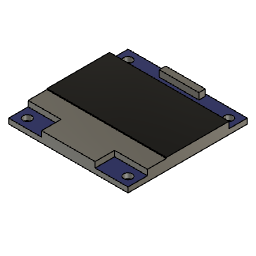
Enclosure_2_v72 (Autodesk Fusion 360 archive; units mm, degrees)
design "OLED"
Autodesk Fusion 360 part; units mm, degrees
sketch "Sketch1" plane through (0, 0, 0) normal (0, 0, 1) x (1, 0, 0)
  line L0 (0, 0) -> (27.85, 0)
  line L1 (27.85, 0) -> (27.85, 27.85)
  line L2 (27.85, 27.85) -> (0, 27.85)
  line L3 (0, 27.85) -> (0, 0)
  dimension "d1" = 27.85
  dimension "d2" = 27.85
  constraint horizontal L0
  constraint vertical L1
  constraint horizontal L2
  constraint vertical L3
  constraint coincident L0.start L3.end
  measures "d1" distance of L0.start L0.end
  measures "d2" distance of L0.start L2.end
extrude "Extrude1" add sketch "Sketch1" along normal blind 1.2
sketch "Sketch2" plane through (0, 0, 1.2) normal (0, 0, 1) x (-1, 0, 0)
  line L0 (0, -27.85) -> (0, 0)
  line L1 (0, 0) -> (-27.85, 0)
  line L2 (-27.85, 0) -> (-27.85, -27.85)
  line L3 (-27.85, -27.85) -> (0, -27.85)
  circle A0 centre (-2.175, -25.675) radius 1
  circle A1 centre (-2.175, -2.175) radius 1
  circle A2 centre (-25.675, -25.675) radius 1
  circle A3 centre (-25.675, -2.175) radius 1
  line L4 (0, -24.675) -> (-27.85, -24.675) construction
  line L5 (0, -3.175) -> (-27.85, -3.175) construction
  line L6 (-24.675, 0) -> (-24.675, -27.85) construction
  line L7 (-3.175, 0) -> (-3.175, -27.85) construction
  line L8 (-24.675, -13.925) -> (-27.85, -13.925) construction
  line L9 (-3.175, -13.925) -> (0, -13.925) construction
  line L10 (-13.925, -24.675) -> (-13.925, -27.85) construction
  line L11 (-13.925, -3.175) -> (-13.925, 0) construction
  dimension "d5" = 2
  dimension "d6" = 21.5
  dimension "d7" = 21.5
  constraint coincident L0 L4.start
  constraint coincident L2 L4.end
  constraint perpendicular L2 L4
  constraint coincident L0 L5.start
  constraint coincident L2 L5.end
  constraint perpendicular L2 L5
  constraint coincident L1 L6.start
  constraint coincident L3 L6.end
  constraint perpendicular L3 L6
  constraint coincident L1 L7.start
  constraint coincident L3 L7.end
  constraint perpendicular L3 L7
  constraint equal A0 A2
  constraint equal A0 A1
  constraint equal A0 A3
  constraint tangent A0 L4
  constraint tangent A0 L7
  constraint tangent A1 L7
  constraint tangent A1 L5
  constraint tangent A3 L5
  constraint tangent A3 L6
  constraint tangent A2 L4
  constraint tangent A2 L6
  constraint midpoint L6 L8.start
  constraint midpoint L2 L8.end
  constraint midpoint L7 L9.start
  constraint midpoint L0 L9.end
  constraint midpoint L4 L10.start
  constraint midpoint L3 L10.end
  constraint midpoint L5 L11.start
  constraint midpoint L1 L11.end
  constraint equal L8 L9
  constraint equal L10 L11
  measures "d5" diameter of A0
  measures "d6" distance of L4 L5
  measures "d7" distance of L6 L7
extrude "Extrude2" cut sketch "Sketch2" against normal through all contours A0 | A1 | A2 | A3
sketch "Sketch3" plane through (0, 0, 1.2) normal (0, 0, 1) x (-1, 0, 0)
  circle A0 centre (-25.675, -2.175) radius 1
  circle A1 centre (-25.675, -25.675) radius 1
  circle A2 centre (-2.175, -2.175) radius 1
  circle A3 centre (-2.175, -25.675) radius 1
  line L0 (0, -27.85) -> (0, 0)
  line L1 (0, 0) -> (-27.85, 0)
  line L2 (-27.85, 0) -> (-27.85, -27.85)
  line L3 (-27.85, -27.85) -> (0, -27.85)
  line L4 (0, -23.55) -> (-27.85, -23.55)
  line L5 (-27.85, -23.55) -> (-27.85, -4.55)
  line L6 (-27.85, -4.55) -> (0, -4.55)
  line L7 (0, -4.55) -> (0, -23.55)
  line L8 (-7.675, -4.55) -> (-20.175, -4.55)
  line L9 (-20.175, -4.55) -> (-20.175, 0)
  line L10 (-20.175, 0) -> (-7.675, 0)
  line L11 (-7.675, 0) -> (-7.675, -4.55)
  line L12 (-13.925, 0) -> (-13.925, -4.55) construction
  dimension "d9" = 19
  dimension "d10" = 4.3
  dimension "d13" = 12.5
  constraint horizontal L4
  constraint vertical L5
  constraint horizontal L6
  constraint vertical L7
  constraint coincident L2 L5.end
  constraint coincident L0 L4.start
  constraint horizontal L8
  constraint vertical L9
  constraint horizontal L10
  constraint vertical L11
  constraint coincident L1 L9.end
  constraint coincident L6 L8.start
  constraint midpoint L10 L12.start
  constraint midpoint L6 L12.end
  constraint vertical L12
  measures "d9" distance of L4 L6
  measures "d10" distance of L3 L4
  measures "d13" distance of L9.end L10.end
extrude "Extrude3" add sketch "Sketch3" along normal blind 1.5 contours L0 L2 L4 L5 L6 L7 L8
extrude "Extrude4" add sketch "Sketch3" along normal blind 1.3 contours L1 L6 L8 L9 L10 L11
sketch "Sketch4" plane through (0, 0, 1.2) normal (0, 0, 1) x (-1, 0, 0)
  line L0 (0, -23.55) -> (-27.85, -23.55)
  line L1 (-27.85, -23.55) -> (-27.85, -27.85)
  line L2 (-27.85, -27.85) -> (0, -27.85)
  line L3 (0, -27.85) -> (0, -23.55)
  circle A0 centre (-25.675, -25.675) radius 1
  circle A1 centre (-2.175, -25.675) radius 1
  line L4 (-9.3, -27.35) -> (-18.55, -27.35)
  line L5 (-18.55, -27.35) -> (-18.55, -25.85)
  line L6 (-18.55, -25.85) -> (-9.3, -25.85)
  line L7 (-9.3, -25.85) -> (-9.3, -27.35)
  line L8 (-13.925, -27.85) -> (-13.925, -27.35) construction
  dimension "d16" = 2
  dimension "d17" = 1.5
  dimension "d18" = 9.25
  constraint horizontal L4
  constraint vertical L5
  constraint horizontal L6
  constraint vertical L7
  constraint midpoint L2 L8.start
  constraint midpoint L4 L8.end
  constraint vertical L8
  measures "d16" distance of L2 L6
  measures "d17" distance of L4.start L6.end
  measures "d18" distance of L4.start L4.end
extrude "Extrude5" add sketch "Sketch4" along normal blind 1.5 contours L4 L5 L6 L7
extrude "Extrude6" add 1 faces at (15.4667, 26.35, 2.7) along direction (0, 0, -1) blind 7
sketch "Sketch5" plane through (0, 25.85, 0) normal (0, -1, 0) x (1, 0, 0)
  line L0 (18.55, 0) -> (9.3, 0)
  line L1 (9.3, 0) -> (9.3, -4.3)
  line L2 (9.3, -4.3) -> (18.55, -4.3)
  line L3 (18.55, -4.3) -> (18.55, 0)
  line L4 (9.3, -2.8) -> (18.55, -2.8)
  dimension "d23" = 1.5
  constraint coincident L1 L4.start
  constraint coincident L3 L4.end
  constraint perpendicular L3 L4
  measures "d23" distance of L2 L4
extrude "Extrude7" add sketch "Sketch5" along normal blind 4 contours L1 L2 L3 L4
sketch "Sketch6" plane through (0, 0, 2.7) normal (0, 0, 1) x (-1, 0, 0)
  line L0 (0, -4.55) -> (-27.85, -4.55)
  line L1 (-27.85, -4.55) -> (-27.85, -23.55)
  line L2 (-27.85, -23.55) -> (0, -23.55)
  line L3 (0, -23.55) -> (0, -4.55)
  line L4 (0, -8.95) -> (-27.85, -8.95)
  dimension "d26" = 14.6
  constraint coincident L3 L4.start
  constraint coincident L1 L4.end
  constraint perpendicular L1 L4
  measures "d26" distance of L2 L4
extrude "Extrude8" cut sketch "Sketch6" against normal up to surface (0.2 mm away) contours L0 L1 L3 L4
